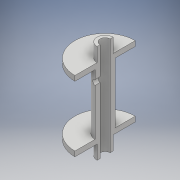
# Autodesk Inventor part: spool
Saved by Autodesk Inventor 2017 (Build 210142000, 142)
## iProperties
Created: 2017-04-28
Part Number: spool
Material: Generic
Document SubType Name: Modeling
Designer: s4321966
Density: 1 g/cm^3
Appearance: Default
Author: s4321966
Autodesk Inventor part; units mm, degrees
ref_plane "YZ Plane" through (0, 0, 0) normal (1, 0, 0) x (0, 1, 0)
ref_plane "XZ Plane" through (0, 0, 0) normal (0, 1, 0) x (-1, 0, 0)
ref_plane "XY Plane" through (0, 0, 0) normal (0, 0, 1) x (1, 0, 0)
sketch "Sketch1" plane through (0, 0, 0) normal (0, 1, 0) x (-1, 0, 0)
  line L0 (0, 0) -> (2.5, 0)
  line L1 (2.5, 0) -> (2.5, -7)
  line L2 (0, 0) -> (4, 0)
  line L3 (4, 0) -> (4, -7)
  line L4 (2.5, -7) -> (4, -7)
  line L5 (4, -7) -> (4, 0)
  line L6 (4, 0) -> (2.5, 0)
  line L7 (2.5, 0) -> (2.5, -7)
  line L8 (2.5, -7) -> (15, -7)
  line L9 (15, -7) -> (15, -9.5)
  line L10 (15, -9.5) -> (2.5, -9.5)
  line L11 (2.5, -9.5) -> (2.5, -7)
  line L12 (2.5, -9.5) -> (5, -9.5)
  line L13 (5, -9.5) -> (5, -39.5)
  line L14 (5, -39.5) -> (2.5, -39.5)
  line L15 (2.5, -39.5) -> (2.5, -9.5)
  line L16 (5, -24.5) -> (-8.9655, -24.5)
  line L17 (0, -49) -> (2.5, -49)
  line L18 (2.5, -49) -> (2.5, -42)
  line L19 (0, -49) -> (4, -49)
  line L20 (4, -49) -> (4, -42)
  line L21 (2.5, -42) -> (4, -42)
  line L22 (4, -42) -> (4, -49)
  line L23 (4, -49) -> (2.5, -49)
  line L24 (2.5, -49) -> (2.5, -42)
  line L25 (2.5, -42) -> (15, -42)
  line L26 (15, -42) -> (15, -39.5)
  line L27 (15, -39.5) -> (2.5, -39.5)
  line L28 (2.5, -39.5) -> (2.5, -42)
  line L29 (2.5, -39.5) -> (5, -39.5)
  line L30 (0, 0) -> (0, -54.8818)
  dimension "d0" = 2.5
  dimension "d1" = 7
  dimension "d2" = 90
  dimension "d3" = 4
  dimension "d4" = 12.5
  dimension "d5" = 2.5
  dimension "d6" = 2.5
  dimension "d7" = 30
  constraints: 62 end point, 9 symmetric about line, 6 horizontal, 6 parallel, 5 perpendicular, 1 midpoint, 1 vertical
  measures "d0" distance of L0.start L0.end
  measures "d1" distance of L0.end L1.end
  measures "d2" angle of L0 L1
  measures "d3" distance of L0.start L2.end
  measures "d4" distance of L9.end L10.end
  measures "d5" distance of L8.end L9.end
  measures "d6" distance of L13.end L14.end
  measures "d7" distance of L12.end L13.end
revolve "Revolution1" add sketch "Sketch1" angle 360 about axis through (0, 0, 0) along (0, 0, -1) contours L2 L3 L4 L1 | L4 L8 L9 L10 L11 | L16 L13 L14 L15 | L15 L10 L13 L16 | L14 L27 L26 L25 L21 L28 | L18 L21 L20 L19
sketch "Sketch2" plane through (0, 0, 0) normal (0, 1, 0) x (-1, 0, 0)
  line L0 (0, 0) -> (0, -15)
  line L1 (0, 0) -> (15, 0) construction
  circle A0 centre (0, -15) radius 1.25
  dimension "d9" = 15
  dimension "d10" = 90
  dimension "d11" = 2.5
  constraints: 4 end point, 1 centre point, 1 coincident, 1 horizontal, 1 perpendicular, 1 vertical
  measures "d9" distance of L0.start L0.end
  measures "d10" angle of L0 L1
  measures "d11" diameter of A0
extrude "Extrusion1" cut sketch "Sketch2" against normal blind 10
sketch "Sketch3" plane through (0, 0, 0) normal (0, 0, 1) x (1, 0, 0)
  circle A0 centre (0, 0) radius 4 projected
  line L0 (0, 0) -> (24.6363, 0)
  line L1 (24.6363, 0) -> (24.6363, -18.6963)
  line L2 (24.6363, -18.6963) -> (0, -18.6963)
  line L3 (0, -18.6963) -> (0, 0)
  line L4 (0, 0) -> (27.3141, 0)
  line L5 (27.3141, 0) -> (27.3141, 19.6701)
  line L6 (27.3141, 19.6701) -> (0, 19.6701)
  line L7 (0, 19.6701) -> (0, 0)
  constraints: 16 end point, 4 parallel, 2 horizontal, 2 perpendicular
extrude "Extrusion2" cut sketch "Sketch3" against normal blind 100 contours L0 L7 A0 | L0 L1 L2 L3 A0 | A0 L3 L0 | A0 L7 L6 L5 L4 L0
body "Solid1"
